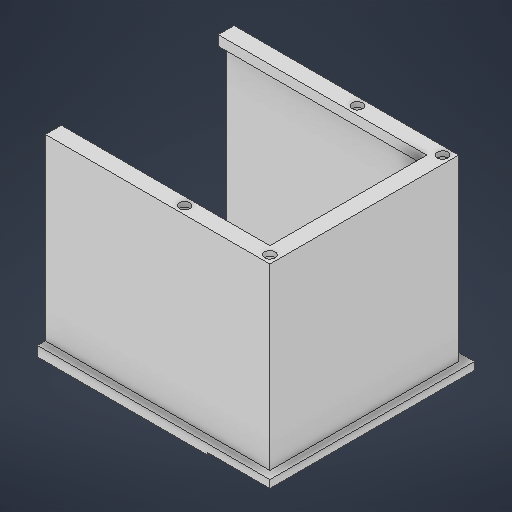
# Autodesk Inventor part: Galvo Housing-01
Saved by Autodesk Inventor 2025 (Build 290162000, 162)
## iProperties
Created: 2024-06-12
Part Number: Galvo Housing-01
Material: Generic
Document SubType Name: Modeling
Designer: mayhe
Density: 1 g/cm^3
Appearance: Default
Author: mayhe
Autodesk Inventor part; units mm, degrees
ref_plane "YZ Plane" through (0, 0, 0) normal (1, 0, 0) x (0, 1, 0)
ref_plane "XZ Plane" through (0, 0, 0) normal (0, 1, 0) x (-1, 0, 0)
ref_plane "XY Plane" through (0, 0, 0) normal (0, 0, 1) x (1, 0, 0)
sketch "Sketch8" plane through (0, 0, 0) normal (0, 1, 0) x (-1, 0, 0)
  line L0 (-56.5, -47.5) -> (56.5, -47.5)
  line L1 (56.5, -47.5) -> (56.5, 47.5)
  line L2 (56.5, 47.5) -> (-56.5, 47.5)
  line L3 (-56.5, 47.5) -> (-56.5, -47.5)
  line L4 (-56.5, -47.5) -> (56.5, 47.5) construction
  line L5 (56.5, -47.5) -> (-56.5, 47.5) construction
  point P0 (0, 0)
  dimension "d26" = 113
  dimension "d27" = 95
  constraints: 12 end point, 2 midpoint, 2 parallel, 1 horizontal, 1 perpendicular
  measures "d26" distance of L2.end L1.end
  measures "d27" distance of L1.end L0.end
extrude "Extrusion7" add sketch "Sketch8" along normal blind 95
sketch "Sketch9" plane through (0, 0, 0) normal (0, -1, 0) x (1, 0, 0)
  line L0 (-56.5, 47.5) -> (56.5, 47.5) projected
  line L1 (-56.5, -47.5) -> (56.5, -47.5)
  line L2 (56.5, -47.5) -> (56.5, 47.5)
  line L3 (56.5, 47.5) -> (-56.5, 47.5)
  line L4 (-56.5, 47.5) -> (-56.5, -47.5)
  line L5 (-56.5, -47.5) -> (56.5, 47.5) construction
  line L6 (56.5, -47.5) -> (-56.5, 47.5) construction
  line L7 (52.5, 43.5) -> (52.5, -43.5)
  line L8 (52.5, -43.5) -> (-56.5, -43.5)
  line L9 (-56.5, 43.5) -> (52.5, 43.5)
  line L10 (48.5, -39.5) -> (48.5, 39.5)
  line L11 (48.5, 39.5) -> (-56.5, 39.5)
  line L12 (-56.5, -39.5) -> (48.5, -39.5)
  line L13 (-54.3018, -43.5) -> (-54.3018, -45.6519)
  line L14 (-54.3018, 45.6519) -> (-54.3018, 43.5)
  line L15 (-49.9386, 39.5) -> (-49.9386, 41.9838)
  line L16 (-49.9386, -41.9838) -> (-49.9386, -39.5)
  point P0 (0, 0)
  dimension "d30" = 4
  dimension "d31" = 4
  dimension "d47" = 4
  dimension "d48" = 4
  dimension "d49" = 4
  dimension "d50" = 4
  constraints: 32 end point, 12 point on line, 8 parallel, 3 perpendicular, 2 midpoint, 1 horizontal
  measures "d30" distance between parallel lines of L2 L7
  measures "d31" distance between parallel lines of L7 L10
  measures "d47" distance between parallel lines of L0 L9
  measures "d48" distance between parallel lines of L11 L9
  measures "d49" distance between parallel lines of L1 L8
  measures "d50" distance between parallel lines of L8 L12
extrude "Extrusion8" cut sketch "Sketch9" against normal blind 115 contours L11 L10 L12 L4
extrude "Extrusion9" cut sketch "Sketch9" against normal blind 90 contours L9 L7 L8 L4 L12 L10 L11
sketch "Sketch10" plane through (0, 0, 0) normal (0, -1, 0) x (1, 0, 0)
  line L0 (56.5, -47.5) -> (-56.5, -47.5)
  line L1 (-56.5, -47.5) -> (-56.5, 47.5)
  line L2 (-56.5, 47.5) -> (56.5, 47.5)
  line L3 (56.5, 47.5) -> (56.5, -47.5)
  line L4 (56.5, -47.5) -> (-56.5, 47.5) construction
  line L5 (-56.5, -47.5) -> (56.5, 47.5) construction
  line L6 (-60.5, 51.5) -> (-60.5, -51.5)
  line L7 (-60.5, -51.5) -> (60.5, -51.5)
  line L8 (60.5, -51.5) -> (60.5, 51.5)
  line L9 (60.5, 51.5) -> (-60.5, 51.5)
  line L10 (-56.5, 47.5) -> (-60.5, 47.5)
  line L11 (-56.5, -47.5) -> (-60.5, -47.5)
  line L12 (-56.5, 47.5) -> (-56.5, 51.5)
  line L13 (-56.5, -47.5) -> (-56.5, -51.5)
  point P0 (0, 0)
  dimension "d36" = 4
  constraints: 28 end point, 5 perpendicular, 5 point on line, 4 parallel, 2 midpoint, 1 horizontal, 3 other
  measures "d36" distance between parallel lines of L1 L6
extrude "Extrusion10" add sketch "Sketch10" against normal blind 5 contours L3 L2 L12 L9 L8 L7 L13 L0
sketch "Sketch11" plane through (0, 0, 0) normal (0, -1, 0) x (1, 0, 0)
  circle A0 centre (-75.5, 17.5) radius 135
  line L0 (52.5, 43.5) -> (52.5, -43.5) projected
  line L1 (60.5, -51.5) -> (60.5, 51.5) projected
  circle A1 centre (-75.5, 17.5) radius 110
  line L2 (10.168, -51.5) -> (60.5, -51.5)
  line L3 (60.5, -51.5) -> (60.5, 51.5)
  line L4 (60.5, 51.5) -> (29.1136, 51.5)
  line L5 (-56.5, 51.5) -> (60.5, 51.5) projected
  point P0 (0, 0)
  dimension "d39" = 270
  dimension "d41" = 136
  dimension "d42" = 220
  constraints: 6 end point, 2 centre point, 2 point on circle, 1 coincident, 1 collinear, 1 perpendicular, 1 point on line
  measures "d39" diameter of A0
  measures "d41" distance from line of L1 A0.centre
  measures "d42" diameter of A1
extrude "Extrusion11" cut sketch "Sketch11" against normal blind 1.125 contours A0 L2 A1 L4 | A0 L4 L1 L2 picked at (50.9054, 12.6578)
sketch "Sketch12" plane through (0, 95, 0) normal (0, 1, 0) x (1, 0, 0)
  line L0 (-56.5, -43.5) -> (52.5, -43.5) projected
  circle A0 centre (52.5, -43.5) radius 2.625
  line L1 (52.5, 43.5) -> (52.5, -43.5) projected
  circle A1 centre (52.5, 43.5) radius 2.625
  line L2 (52.5, 43.5) -> (-56.5, 43.5) projected
  circle A2 centre (9.525, 43.5) radius 2.625
  circle A3 centre (9.525, -43.5) radius 2.625
  point P0 (0, 0)
  dimension "d51" = 5.25
  dimension "d52" = 5.25
  dimension "d53" = 5.25
  dimension "d54" = 5.25
  constraints: 4 centre point, 1 point on line
  measures "d51" diameter of A0
  measures "d52" diameter of A1
  measures "d53" diameter of A2
  measures "d54" diameter of A3
extrude "Extrusion13" cut sketch "Sketch12" against normal blind 2.5
body "Solid3"
